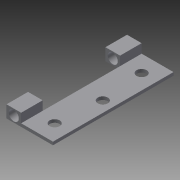
# Autodesk Inventor part: door hinge for conveyor
Saved by Autodesk Inventor 2015 (Build 190159000, 159)
## iProperties
Created: 2015-02-03
Part Number: door hinge for conveyor
Material: Generic
Document SubType Name: Modeling
Designer: szymsea16
Density: 1 g/cm^3
Appearance: Default
Author: szymsea16
Autodesk Inventor part; units mm, degrees
ref_plane "YZ Plane" through (0, 0, 0) normal (1, 0, 0) x (0, 1, 0)
ref_plane "XZ Plane" through (0, 0, 0) normal (0, 1, 0) x (-1, 0, 0)
ref_plane "XY Plane" through (0, 0, 0) normal (0, 0, 1) x (1, 0, 0)
sketch "Sketch1" plane through (0, 0, 0) normal (0, 1, 0) x (-1, 0, 0)
  line L0 (0, 0) -> (0, -63.881)
  line L1 (0, -63.881) -> (16.891, -63.881)
  line L2 (16.891, -63.881) -> (16.891, 0)
  line L3 (16.891, 0) -> (0, 0)
  line L4 (16.891, 0) -> (24.638, 0)
  line L5 (24.638, 0) -> (24.638, -11.43)
  line L6 (24.638, -11.43) -> (16.891, -11.43)
  line L7 (16.891, -63.881) -> (24.638, -63.881)
  line L8 (24.638, -63.881) -> (24.638, -52.451)
  line L9 (24.638, -52.451) -> (16.891, -52.451)
  dimension "d0" = 63.881
  dimension "d1" = 16.891
  dimension "d2" = 7.747
  dimension "d3" = 11.43
  dimension "d4" = 7.747
  dimension "d5" = 11.43
  constraints: 20 end point, 6 perpendicular, 5 point on line, 1 vertical
  measures "d0" distance of L0.start L0.end
  measures "d1" distance of L0.end L1.end
  measures "d2" distance of L2.end L4.end
  measures "d3" distance of L4.end L5.end
  measures "d4" distance of L1.end L7.end
  measures "d5" distance of L7.end L8.end
extrude "Extrusion1" add sketch "Sketch1" along normal blind 1.651 contours L3 L2 L1 L0
extrude "Extrusion2" add sketch "Sketch1" along normal blind 6.477 contours L4 L5 L6 L2
extrude "Extrusion3" add sketch "Sketch1" along normal blind 6.477 contours L2 L9 L8 L7
hole "Hole1" at (-8.001, 1.651, -8.89) direction (0, -1, 0) diameter 5.334 end through all
hole "Hole2" at (-8.001, 1.651, -54.991) direction (0, -1, 0) diameter 5.334 end through all
hole "Hole3" at (-5.715, 1.651, -32.131) direction (0, -1, 0) diameter 5.334 end through all
hole "Hole4" at (-20.7645, 3.2385, 0) direction (0, 0, -1) diameter 5.334 end through all
body "Solid1"
